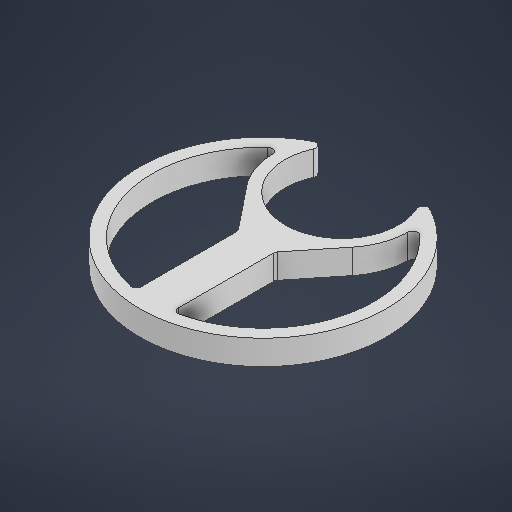
# Autodesk Inventor part: Gear Holder 1
Saved by Autodesk Inventor 2026.2 (Build 302298000, 298)
## iProperties
Created: 2026-01-26
Part Number: Gear Holder 1
Material: Generic
Document SubType Name: Modeling
Designer: Cobble
Density: 1 g/cm^3
Appearance: Default
Author: Cobble
Autodesk Inventor part; units mm, degrees
ref_plane "YZ Plane" through (0, 0, 0) normal (1, 0, 0) x (0, 1, 0)
ref_plane "XZ Plane" through (0, 0, 0) normal (0, 1, 0) x (-1, 0, 0)
ref_plane "XY Plane" through (0, 0, 0) normal (0, 0, 1) x (1, 0, 0)
sketch "Sketch1" plane through (0, 0, 0) normal (0, 0, 1) x (1, 0, 0)
  circle A0 centre (0, 0) radius 60.5521
  arc A1 (-0.7258, 10.3355) -> (0.2666, 10.325) centre (0, 32) ccw
  circle A2 centre (0, 0) radius 60.5521
  circle A3 centre (0, 32) radius 2.5
  circle A4 centre (0, 0) radius 50
  circle A5 centre (0, 0) radius 57.5
  circle A6 centre (0, 0) radius 57
  circle A7 centre (0, 0) radius 7.5
  circle A8 centre (0, 32) radius 23
  circle A9 centre (0, 0) radius 45
  circle A10 centre (0, 32) radius 27.5
  line L0 (-5.8547, -4.6875) -> (-21.4672, 14.8125)
  line L1 (5.8547, -4.6875) -> (21.4672, 14.8125)
  line L2 (0, 0) -> (0, 32)
  line L3 (7.5, 44.3706) -> (7.5, -44.3706)
  line L4 (-7.5, 44.3706) -> (-7.5, -44.3706)
  point P0 (27.2328, 35.8242)
  point P1 (7.5, -2.6325)
  point P2 (-27.2328, 35.8242)
  point P3 (-7.5, -2.6325)
  point P4 (17.6083, 46.7969)
  point P5 (-17.6083, 46.7969)
  dimension "d0" = 5
  dimension "d1" = 100
  dimension "d2" = 115
  dimension "d4" = 15
  dimension "d5" = 46
  dimension "d6" = 90
  dimension "d7" = 55
  dimension "d8" = 32
  constraints: 11 centre point, 10 coincident, 10 end point, 10 point on circle, 6 tangent, 2 vertical, 1 concentric, 1 parallel
  measures "d0" diameter of A3
  measures "d1" diameter of A4
  measures "d2" diameter of A5
  measures "d4" diameter of A7
  measures "d5" diameter of A8
  measures "d6" diameter of A9
  measures "d7" diameter of A10
  measures "d8" distance of A1.centre A0.centre
extrude "Extrusion1" add sketch "Sketch1" along normal blind 10 contours A4 A10 A9 | A10 A9 A8 A4 | A4 A8 A9 A10 | A10 L3 A8 A9 | A9 A8 L4 A10 | L4 L0 A7 L1 L3 A9 | A10 L4 L0 | L1 L3 A10 | A8 L2 A7 A10 L4 | L4 A7 L0 | A10 A7 L4 | L3 A10 A7 L2 A8 | L1 A7 L3 | L3 A7 A10 | A7 A10 | A7 L2 A10 | A10 L2 A7
fillet "Fillet1" radius 2 8 edges at (-17.6083, 46.7969, 5) (17.6083, 46.7969, 5) (27.2328, 35.8242, 5) (-27.2328, 35.8242, 5) (-7.5, -2.6325, 5) (7.5, -2.6325, 5) (7.5, -44.3706, 5) (-7.5, -44.3706, 5)
body "Solid1"
